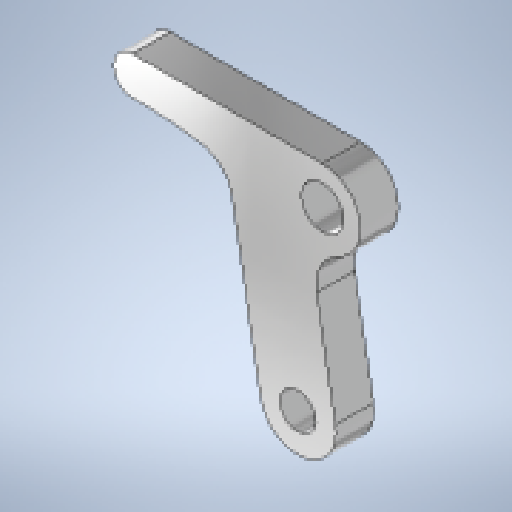
# Autodesk Inventor part: Lever
Saved by Autodesk Inventor 2023.2 (Build 272271000, 271)
## iProperties
Created: 2024-02-17
Part Number: Lever
Material: Aluminum 6061
Document SubType Name: Modeling
Designer: Nathan Cai
Density: 2.7 g/cm^3
Appearance: Aluminum - Flat
Author: Nathan Cai
Autodesk Inventor part; units mm, degrees
ref_plane "YZ Plane" through (0, 0, 0) normal (1, 0, 0) x (0, 1, 0)
ref_plane "XZ Plane" through (0, 0, 0) normal (0, 1, 0) x (-1, 0, 0)
ref_plane "XY Plane" through (0, 0, 0) normal (0, 0, 1) x (1, 0, 0)
sketch "Sketch1" plane through (0, 0, 0) normal (0, 0, 1) x (1, 0, 0)
  circle A0 centre (0, 0) radius 1.778
  circle A1 centre (0, 0) radius 3.175
  line L0 (0, 0) -> (-15.875, 0) construction
  circle A2 centre (-2.0605, -15.7407) radius 3.175
  circle A3 centre (-2.0605, -15.7407) radius 5 construction
  circle A4 centre (-2.0605, -15.7407) radius 1.5
  line L1 (0, 0) -> (-2.0605, -15.7407) construction
  line L2 (-2.0605, -15.7407) -> (-3.5478, -15.546) construction
  line L3 (0, 0) -> (-2.0605, -15.7407) construction
  arc A5 (-5.1273, -14.919) -> (1.0064, -16.5625) centre (-2.0605, -15.7407) ccw
  arc A6 (-1.2212, -2.9308) -> (-15.875, 0) centre (-15.875, -38.1) ccw
  arc A7 (-15.875, 3.175) -> (-15.875, 0) centre (-15.875, 1.5875) ccw
  line L4 (-15.875, 3.175) -> (0, 3.175)
  line L5 (-2.0605, -15.7407) -> (-4.836, 0) construction
  line L6 (1.0663, -15.1894) -> (-1.7092, 0.5513)
  line L7 (-7.9627, -0.5513) -> (-5.1872, -16.292)
  arc A8 (-5.1872, -16.292) -> (1.0663, -15.1894) centre (-2.0605, -15.7407) ccw
  arc A9 (-1.7092, 0.5513) -> (-7.9627, -0.5513) centre (-4.836, 0) ccw
  circle A10 centre (6.7469, -0.7937) radius 3.175
  circle A11 centre (6.7469, -0.7937) radius 1.5
  line L8 (7.1178, 2.3595) -> (0.371, 3.1533)
  arc A12 (4.769, -3.2774) -> (-0.4834, -6.4004) centre (2.7339, -5.8331) ccw
  circle A13 centre (6.7469, -0.7937) radius 5 construction
  point P0 (0, 3.175)
  point P1 (-7.9116, -0.8415)
  point P2 (-5.1872, -16.292)
  point P3 (1.0663, -15.1894)
  point P4 (-1.0859, -2.9835)
  point P5 (-2.418, 2.0577)
  point P6 (0.6312, -3.1116)
  point P7 (1.3474, -2.8749)
  point P8 (-1.4243, -1.0642)
  point P9 (-1.7024, 0.5129)
  dimension "d24" = 3
  dimension "d0" = 3.556
  dimension "d1" = 6.35
  dimension "d9" = 15.875
  dimension "d22" = 6.35
  dimension "d23" = 10
  dimension "d26" = 15.875
  dimension "d29" = 3.175
  dimension "d30" = 6.35
  dimension "d31" = 6.35
  dimension "d32" = 3
  dimension "d36" = 10
  dimension "d37" = 100
  dimension "d38" = 4.7625
  dimension "d39" = 6.7469
  dimension "d40" = 0.7937
  constraints: 22 end point, 16 point on circle, 14 tangent, 13 centre point, 6 coincident, 2 point on line, 1 concentric, 1 horizontal, 1 parallel, 1 perpendicular, 3 other
  measures "d0" diameter of A0
  measures "d1" diameter of A1
  measures "d9" distance of L0.start L0.end
  measures "d22" diameter of A2
  measures "d23" diameter of A3
  measures "d26" distance from line of point (0, 0) L2
  measures "d29" diameter of A7
  measures "d30" diameter of A9
  measures "d31" diameter of A10
  measures "d32" diameter of A11
  measures "d36" diameter of A13
  measures "d37" angle of L0 L5
  measures "d38" distance from line of A0.centre L5
  measures "d39" horizontal distance of A0.centre A11.centre
  measures "d40" vertical distance of A0.centre A11.centre
extrude "Extrusion1" add sketch "Sketch1" along normal blind 3.175 contours A0 L6 A9 A1 | A0 L6 A1 A9 | L6 A2 L7 A6 A1 | A1 A12 L6 | A9 L4 A1 | A1 A6 L7 A9 | A9 L7 A6 A7 L4 | A2
fillet "Fillet1" radius 3.175 1 edges at (-7.9116, -0.8415, 1.5875)
body "Solid1"
